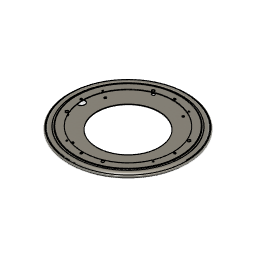
12in lazy susan (Autodesk Fusion 360 design; units mm, degrees)
Autodesk Fusion 360 part; units mm, degrees
sketch "Sketch1" plane through (0, 0, 0) normal (0, 1, 0) x (1, 0, 0)
  circle A0 centre (0, 0) radius 152.4
  circle A1 centre (0, 0) radius 79.375
  line L0 (0, 0) -> (-119.253, 0) construction
  circle A2 centre (-119.253, 0) radius 9.525
  circle A3 centre (-99.4445, 41.3427) radius 2.54
  circle A4 centre (-110.4699, -45.7548) radius 3.6195
  line L1 (0, 0) -> (-99.4445, 41.3427) construction
  line L2 (0, 0) -> (-110.4699, -45.7548) construction
  line L3 (-152.4, 9.525) -> (-152.4, 14.9978)
  line L4 (-152.4, 14.9978) -> (-152.4, -9.525) construction
  line L5 (-152.4, 9.525) -> (-119.253, 9.525) construction
  line L6 (-152.4, -9.525) -> (-119.253, -9.525) construction
  line L7 (-128.778, 9.525) -> (-128.778, -9.525) construction
  line L8 (-98.4694, 43.6881) -> (-139.7483, 60.8492) construction
  line L9 (-139.7483, 60.8492) -> (-141.6984, 56.1585) construction
  line L10 (-141.6984, 56.1585) -> (-100.4196, 38.9973) construction
  line L11 (-100.8148, 44.6632) -> (-102.7649, 39.9724) construction
  line L12 (-142.1858, -54.9734) -> (-139.4157, -61.6614) construction
  line L13 (-139.4157, -61.6614) -> (-109.0849, -49.0989) construction
  line L14 (-142.1858, -54.9734) -> (-111.8549, -42.4108) construction
  line L15 (-115.199, -43.7959) -> (-112.4289, -50.4839) construction
  line L16 (-119.253, 0) -> (-110.4699, -45.7548) construction
  line L17 (-119.253, 0) -> (-99.4445, 41.3427) construction
  circle A5 centre (-41.3427, -99.4445) radius 2.54
  circle A6 centre (0, -119.253) radius 9.525 construction
  circle A7 centre (45.7548, -110.4699) radius 3.6195
  circle A8 centre (99.4445, -41.3427) radius 2.54
  circle A9 centre (119.253, 0) radius 9.525
  circle A10 centre (110.4699, 45.7548) radius 3.6195
  circle A11 centre (41.3427, 99.4445) radius 2.54
  circle A12 centre (0, 119.253) radius 9.525 construction
  circle A13 centre (-45.7548, 110.4699) radius 3.6195
  point P0 (-140.7233, 58.5039)
  point P1 (-140.8007, -58.3174)
  point P2 (-115.1373, 8.5899)
  point P3 (-100.4196, 38.9973)
  point P4 (-117.4574, -9.3542)
  point P5 (-111.8549, -42.4108)
  dimension "d1" = 304.8
  dimension "d2" = 158.75
  dimension "d3" = 19.05
  dimension "d4" = 5.08
  dimension "d5" = 7.239
  dimension "d6" = 23.622
  dimension "d7" = 42.164
  dimension "d8" = 29.21
  dimension "d9" = 33.528
  dimension "d10" = 33.782
  dimension "d12" = 360
  constraint coincident A0.centre A1.centre
  constraint horizontal L0
  constraint coincident L0.end A2.centre
  constraint coincident A3.centre L1.end
  constraint coincident A4.centre L2.end
  constraint vertical L3
  constraint parallel L3 L4
  constraint tangent A0 L4
  constraint coincident A2 L5.end
  constraint tangent A2 L5
  constraint coincident A2 L6.end
  constraint tangent A2 L6
  constraint horizontal L5
  constraint horizontal L6
  constraint coincident L5 L7.start
  constraint perpendicular L6 L7
  constraint coincident L6 L7.end
  constraint tangent A2 L7
  constraint coincident A3 P3
  constraint tangent A3 L10
  constraint coincident A3 L8.start
  constraint tangent A3 L8
  constraint tangent A0 L9
  constraint parallel L1 L8
  constraint parallel L1 L10
  constraint midpoint L9 P0
  constraint coincident A0 P0
  constraint coincident L8 L11.start
  constraint coincident L10 L11.end
  constraint perpendicular L10 L11
  constraint tangent A3 L11
  constraint coincident A4 L13.end
  constraint tangent A4 L13
  constraint coincident A4 P5
  constraint tangent A4 L14
  constraint midpoint L12 P1
  constraint coincident A0 P1
  constraint tangent A0 L12
  constraint parallel L2 L14
  constraint parallel L2 L13
  constraint coincident L14 L15.start
  constraint coincident L13 L15.end
  constraint perpendicular L13 L15
  constraint tangent A4 L15
  constraint coincident L17 P2
  constraint coincident A2 P2
  constraint coincident P3 L10.end
  constraint coincident A2 P4
  constraint coincident L16 P4
  constraint coincident P5 L14.end
  measures "d1" diameter of A0
  measures "d2" diameter of A1
  measures "d3" diameter of A2
  measures "d4" diameter of A3
  measures "d5" diameter of A4
  measures "d6" distance of L4 L7
  measures "d7" distance of P0 L11
  measures "d8" distance of P1 L15
  measures "d9" distance of P4 P5
  measures "d10" distance of P2 P3
extrude "Extrude1" add sketch "Sketch1" along normal blind 6.096 makes body 1
sketch "Sketch2" plane through (0, 0, 0) normal (0, 0, 1) x (1, 0, 0)
  line L0 (152.4, 6.096) -> (-152.4, 6.096)
  line L1 (152.4, 0) -> (-152.4, 0)
  circle A0 centre (149.352, 3.048) radius 3.048
  line L2 (152.4, 6.096) -> (152.4, 0)
  line L3 (146.304, 0) -> (146.304, 3.048)
  line L4 (146.304, 1.27) -> (0, 1.27)
  line L5 (0, 1.27) -> (0, 0)
  line L6 (0, 1.27) -> (0, 6.096)
  line L7 (146.304, 1.27) -> (149.352, 1.27)
  arc A1 (149.352, 1.27) -> (149.352, 4.826) centre (149.352, 3.048) ccw
  arc A2 (149.352, 6.096) -> (149.352, 4.826) centre (149.352, 5.461) ccw
  line L8 (149.352, 6.096) -> (149.352, 4.826) construction
  dimension "d15" = 1.27
  constraint coincident L0.start L2.start
  constraint coincident L1.start L2.end
  constraint tangent A0 L2
  constraint tangent L0 A0
  constraint tangent L1 A0
  constraint coincident L1 L3.start
  constraint perpendicular L0 L3
  constraint tangent A0 L3
  constraint coincident A0 L3.end
  constraint coincident L3 L4.start
  constraint perpendicular L3 L4
  constraint coincident L5.end origin
  constraint vertical L5
  constraint midpoint L0 L6.end
  constraint perpendicular L3 L7
  constraint tangent L7 A1
  constraint coincident L0 A2.start
  constraint coincident A0 A2.start
  constraint tangent A1 A2
  constraint concentric A0 A1
  constraint vertical L8
  measures "d15" distance of L1 L4
revolve "Revolve1" cut sketch "Sketch2" angle 360 about axis through (0, 0, 0) along (0, -1, 0) contours L0 A0 L2 | L0 A0 L3 L4 L6 | A0 L7 A1 A2 | L1 A0 L2 | A0 L3 L7 picked at (148.2442, 3.069) bodies 1
sketch "Sketch3" plane through (0, 0, 0) normal (0, 0, 1) x (1, 0, 0)
  line L0 (79.375, 1.27) -> (-79.375, 1.27)
  line L1 (-109.728, 1.27) -> (-128.778, 1.27)
  line L2 (-96.9045, 1.27) -> (-101.9845, 1.27)
  line L3 (-106.8504, 1.27) -> (-114.0894, 1.27)
  line L4 (-38.8027, 1.27) -> (-43.8827, 1.27)
  line L5 (49.3743, 1.27) -> (42.1353, 1.27)
  line L6 (101.9845, 1.27) -> (96.9045, 1.27)
  line L7 (128.778, 1.27) -> (109.728, 1.27)
  line L8 (114.0894, 1.27) -> (106.8504, 1.27)
  line L9 (-42.1353, 1.27) -> (-49.3743, 1.27)
  line L10 (43.8827, 1.27) -> (38.8027, 1.27)
  line L11 (-149.352, 1.27) -> (149.352, 1.27)
  line L12 (-149.352, 4.826) -> (149.352, 4.826)
  line L13 (-149.352, 1.27) -> (149.352, 1.27)
  line L14 (-149.352, 0) -> (149.352, 0)
  line L15 (149.352, 6.096) -> (-149.352, 6.096)
  arc A0 (149.352, 1.27) -> (149.352, 4.826) centre (149.352, 3.048) ccw
  arc A1 (149.352, 0) -> (149.352, 6.096) centre (149.352, 3.048) ccw
  circle A2 centre (149.352, 3.048) radius 1.5
  arc A3 (149.352, 6.096) -> (149.352, 4.826) centre (149.352, 5.461) ccw
  line L16 (114.3, 1.27) -> (114.3, 6.096) construction
  line L17 (133.35, 8.89) -> (114.935, 8.89)
  arc A4 (114.935, 8.89) -> (114.935, 7.62) centre (114.935, 8.255) ccw
  line L18 (114.935, 7.62) -> (133.35, 7.62)
  line L19 (133.35, 8.89) -> (133.35, 7.62) construction
  arc A5 (133.35, 8.89) -> (136.9485, 7.6531) centre (135.6764, 9.8053) ccw
  arc A6 (148.7789, 5.0638) -> (136.9485, 7.6531) centre (141.472, 0) ccw
  line L20 (133.35, 8.89) -> (141.472, 8.89) construction
  line L21 (149.9719, 4.4139) -> (149.0638, 4.826)
  arc A7 (148.7789, 5.0638) -> (149.0638, 4.826) centre (149.352, 5.461) ccw
  arc A8 (133.35, 7.62) -> (137.3861, 6.7496) centre (135.8289, 9.3219) ccw
  arc A9 (147.9569, 4.4942) -> (137.3861, 6.7496) centre (141.472, 0) ccw
  arc A10 (147.9569, 4.4942) -> (148.3067, 4.1238) centre (149.352, 5.461) ccw
  arc A11 (147.86, 3.2023) -> (146.9641, 5.6647) centre (144.8759, 3.5108) ccw
  dimension "d17" = 3
  dimension "d18" = 114.3
  dimension "d19" = 8.89
  dimension "d20" = 1.27
  dimension "d21" = 1.27
  dimension "d22" = 19.05
  dimension "d23" = 8.89
  dimension "d24" = 2.5
  dimension "d25" = 1
  dimension "d26" = 3
  constraint tangent L12 A0
  constraint coincident L11.end L13.end
  constraint coincident L12.end A0.end
  constraint tangent L14 A1
  constraint coincident L14.end A1.start
  constraint coincident L15.start A1.end
  constraint concentric A1 A2
  constraint tangent L15 A3
  constraint coincident L7 L16.start
  constraint coincident L15 L16.end
  constraint perpendicular L15 L16
  constraint horizontal L17
  constraint tangent L17 A4
  constraint tangent A4 L18
  constraint parallel L15 L18
  constraint tangent L16 A4
  constraint vertical L19
  constraint tangent A5 A6
  constraint coincident A6 L20.end
  constraint tangent A6 L20
  constraint horizontal L20
  constraint coincident A2 L21.start
  constraint tangent A2 L21
  constraint tangent L21 A7
  constraint tangent A6 A7
  constraint coincident L12 L21.end
  constraint concentric A3 A7
  constraint tangent A5 A8
  constraint tangent A9 A10
  constraint concentric A6 A9
  constraint concentric A7 A10
  constraint coincident A2 A10.end
  constraint tangent A8 A9
  constraint tangent A2 A11
  constraint coincident A2 A11.start
  constraint coincident A9 A11.end
  constraint tangent A9 A11
  measures "d17" diameter of A2
  measures "d18" distance of origin L16
  measures "d19" distance of L14 L17
  measures "d20" distance of L11 L14
  measures "d21" distance of L17 L18
  measures "d22" distance of L16 L17.start
  measures "d23" radius of A6
  measures "d24" radius of A5
  measures "d25" distance of A6 A9
  measures "d26" radius of A11
revolve "Revolve2" add sketch "Sketch3" angle 360 about axis through (0, 1.75, 0) along (0, 1, 0) separate body contours L12 A2 L21 A9 A10 | L12 L15 A6 A7 A9 | L12 A2 A9 A10 A11 | L12 A9 A11 | A2 | L15 L17 A4 L18 A5 A6 A8 A9 makes body 2
fillet "Fillet1" radius 2 1 edges at (-124.3259, 8.89, -48.2214) on bodies 2
sketch "Sketch4" plane through (0, 8.89, 0) normal (0, 1, 0) x (-1, 0, 0)
  circle A0 centre (0, 0) radius 114.935
  circle A1 centre (0, 0) radius 132.2484
  line L0 (0, 0) -> (119.253, 0) construction
  line L1 (0, 0) -> (110.0956, -45.8284) construction
  line L2 (0, 0) -> (110.0956, 45.8284) construction
  circle A2 centre (119.253, 0) radius 9.525
  circle A3 centre (110.0956, -45.8284) radius 1.651
  circle A4 centre (119.253, 0) radius 2.54
  circle A5 centre (110.0956, 45.8284) radius 3.4925
  circle A6 centre (0, 119.253) radius 2.54
  circle A7 centre (45.8284, 110.0956) radius 1.651
  circle A8 centre (-45.8284, 110.0956) radius 3.4925
  circle A9 centre (-119.253, 0) radius 2.54
  circle A10 centre (-110.0956, 45.8284) radius 1.651
  circle A11 centre (-110.0956, -45.8284) radius 3.4925
  circle A12 centre (0, -119.253) radius 2.54
  circle A13 centre (-45.8284, -110.0956) radius 1.651
  circle A14 centre (45.8284, -110.0956) radius 3.4925
  dimension "d30" = 6.985
  dimension "d31" = 5.08
  dimension "d32" = 3.302
  dimension "d33" = 22.6
  dimension "d34" = 22.6
  dimension "d36" = 360
  constraint coincident A0.centre A1.centre
  constraint horizontal L0
  constraint equal L0 L1
  constraint equal L1 L2
  constraint coincident L0.end A2.centre
  constraint coincident L1.end A3.centre
  constraint concentric A2 A4
  constraint coincident L2.end A5.centre
  measures "d30" diameter of A5
  measures "d31" diameter of A4
  measures "d32" diameter of A3
  measures "d33" angle of L0 L1
  measures "d34" angle of L0 L2
extrude "Extrude2" cut sketch "Sketch4" against normal blind 3 contours A3 | A4 | A5 | A6 | A7 | A8 | A9 | A10 | A11 | A12 | A13 | A14 bodies 2
copy_body "Body->Comp1" bodies 1 removing the originals makes body 3 in component "Component"
copy_body "Body->Comp2" bodies 2 removing the originals makes body 4 in component "Component'"
sketch "Sketch5" plane through (0, 0, 0) normal (0, -1, 0) x (1, 0, 0)
  circle A0 centre (0, 0) radius 149.352
  circle A1 centre (110.4699, -45.7548) radius 3.6195
  circle A2 centre (41.3427, -99.4445) radius 2.54
  circle A3 centre (119.253, 0) radius 9.525
  circle A4 centre (-45.7548, -110.4699) radius 3.6195
  circle A5 centre (45.7548, 110.4699) radius 3.6195
  circle A6 centre (-41.3427, 99.4445) radius 2.54
  circle A7 centre (-110.4699, 45.7548) radius 3.6195
  circle A8 centre (-99.4445, -41.3427) radius 2.54
  circle A9 centre (-119.253, 0) radius 9.525
  circle A10 centre (0, 0) radius 79.375
  circle A11 centre (0, 0) radius 260.1473
  curve K0
component "Component" placed x (1, 0, 0) y (0, 1, 0) z (0, 0, 1) at (0, 0, 0)
component "Component'" placed x (1, 0, 0) y (0, 1, 0) z (0, 0, 1) at (0, 0, 0)
equation "d18 = ( 9 in ) / 2"
equation "d33 = ( 22.6 ) * 1 deg"
equation "d34 = d33"
